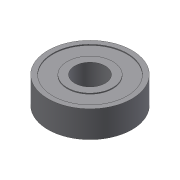
# Autodesk Inventor part: bearing_1
Saved by Autodesk Inventor 2017 (Build 210142000, 142)
## iProperties
Created: 2021-08-28
Part Number: bearing_1
Material: Generic
Document SubType Name: Modeling
Designer: jwoods
Density: 1 g/cm^3
Appearance: Default
Author: jwoods
Autodesk Inventor part; units mm, degrees
ref_plane "YZ Plane" through (0, 0, 0) normal (1, 0, 0) x (0, 1, 0)
ref_plane "XZ Plane" through (0, 0, 0) normal (0, 1, 0) x (-1, 0, 0)
ref_plane "XY Plane" through (0, 0, 0) normal (0, 0, 1) x (1, 0, 0)
sketch "Sketch1" plane through (0, 0, 0) normal (0, 1, 0) x (-1, 0, 0)
  circle A0 centre (0, 0) radius 3.975
  circle A1 centre (0, 0) radius 5.965
  dimension "d0" = 7.95
  dimension "d1" = 11.93
  constraints: 2 centre point, 2 coincident
  measures "d0" diameter of A0
  measures "d1" diameter of A1
extrude "Extrusion1" add sketch "Sketch1" along normal blind 7
sketch "Sketch2" plane through (0, 7, 0) normal (0, 1, 0) x (1, 0, 0)
  circle A0 centre (0, 0) radius 5.965 projected
  circle A1 centre (0, 0) radius 11
  dimension "d4" = 22
  constraints: 1 centre point, 1 coincident
  measures "d4" diameter of A1
extrude "Extrusion2" add sketch "Sketch2" against normal up to surface (7 mm away)
sketch "Sketch3" plane through (0, 0, 0) normal (0, -1, 0) x (1, 0, 0)
  circle A0 centre (0, 0) radius 5.96
  circle A1 centre (0, 0) radius 9.725
  dimension "d7" = 11.92
  dimension "d8" = 19.45
  constraints: 2 centre point, 2 coincident
  measures "d7" diameter of A0
  measures "d8" diameter of A1
extrude "Extrusion3" cut sketch "Sketch3" against normal blind 0.25
sketch "Sketch4" plane through (0, 7, 0) normal (0, 1, 0) x (1, 0, 0)
  circle A0 centre (0, 0) radius 5.96 projected
  circle A1 centre (0, 0) radius 9.725 projected
  circle A2 centre (0, 0) radius 5.96 projected
  circle A3 centre (0, 0) radius 9.725 projected
extrude "Extrusion4" cut sketch "Sketch4" against normal blind 0.25
body "Solid1"
